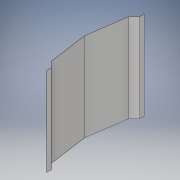
# Autodesk Inventor part: waterbed bottom
Saved by Autodesk Inventor 2019 (Build 230136000, 136)
## iProperties
Created: 2018-08-04
Part Number: waterbed bottom
Material: Generic
Document SubType Name: Sheet Metal
Designer: torba
Density: 1 g/cm^3
Sheet Metal Rule: Default
Appearance: Default
Author: torba
Autodesk Inventor part; units mm, degrees
ref_plane "YZ Plane" through (0, 0, 0) normal (1, 0, 0) x (0, 1, 0)
ref_plane "XZ Plane" through (0, 0, 0) normal (0, 1, 0) x (-1, 0, 0)
ref_plane "XY Plane" through (0, 0, 0) normal (0, 0, 1) x (1, 0, 0)
sketch "Sketch1" plane through (0, 0, 0) normal (0, 1, 0) x (-1, 0, 0)
  line L0 (66.675, 1289.05) -> (142.875, 1212.85)
  line L1 (66.675, 69.85) -> (142.875, 146.05)
  line L2 (66.675, 6.35) -> (66.675, 69.85)
  line L3 (66.675, 1289.05) -> (66.675, 1352.55)
  line L4 (142.875, 1212.85) -> (219.075, 679.45)
  line L5 (219.075, 679.45) -> (142.875, 146.05)
  line L6 (66.675, 1352.55) -> (65.0875, 1352.55)
  line L7 (65.0875, 1352.55) -> (65.0875, 1288.3924)
  line L8 (65.0875, 1288.3924) -> (141.3783, 1212.1016)
  line L9 (141.3783, 1212.1016) -> (217.4714, 679.45)
  line L10 (217.4714, 679.45) -> (141.3783, 146.7984)
  line L11 (141.3783, 146.7984) -> (65.0875, 70.5076)
  line L12 (65.0875, 70.5076) -> (65.0875, 6.35)
  line L13 (65.0875, 6.35) -> (66.675, 6.35)
  point P0 (0, 0)
  dimension "d25" = 163.74
  dimension "d26" = 143.13
  dimension "d27" = 323.2892
  dimension "d28" = 323.2892
  dimension "d29" = 64.6578
  dimension "d30" = 237.0788
  dimension "d31" = 63.5
  dimension "d32" = 63.5
  dimension "d33" = 8.13
  dimension "d34" = 8.13
  dimension "d35" = 312.9619
  dimension "d36" = 120.7844
  dimension "d37" = 1.5875
  dimension "d38" = 1.5875
  dimension "d39" = 1.5875
  dimension "d40" = 1.5875
  dimension "d41" = 1.5875
  dimension "d42" = 1.5875
  constraints: 28 end point, 4 parallel, 3 perpendicular, 1 collinear, 1 horizontal, 1 vertical
  measures "d25" angle of L4 L5
  measures "d26" angle of L4 L0
  measures "d27" distance from line of L4.end L0
  measures "d28" distance from line of L4.end L1
  measures "d29" distance from line of L0.start L4
  measures "d30" distance from line of L1.start L4
  measures "d31" distance of L0.start L3.end
  measures "d32" distance of L2.start L1.start
  measures "d33" angle of L3 L4
  measures "d34" angle of L2 L4
  measures "d35" distance from line of point (0, 0) L4
  measures "d36" distance from line of point (0, 0) L5
  measures "d37" distance of L3.end L6.end
  measures "d38" distance between parallel lines of L8 L0
  measures "d39" distance between parallel lines of L4 L9
  measures "d40" distance between parallel lines of L5 L10
  measures "d41" distance between parallel lines of L1 L11
  measures "d42" distance between parallel lines of L2 L12
extrude "Extrusion1" add sketch "Sketch1" along normal blind 1219.2
equation "\"d38\" = d37"
equation "\"d39\" = d37"
equation "\"d40\" = d37"
equation "\"d41\" = d37"
equation "\"d42\" = d37"
equation "\"BendRadius\" = Thickness"
equation "\"BendReliefWidth\" = Thickness"
equation "\"BendReliefDepth\" = 0.5 * Thickness"
equation "\"CornerReliefSize\" = 4 * Thickness"
equation "\"MinimumRemnant\" = 2 * Thickness"
equation "\"TransitionRadius\" = BendRadius"
equation "\"JacobiRadiusSize\" = Thickness"
equation "\"GapSize\" = Thickness"
equation "\"Thickness\" = 0.5"
body "Solid1"
